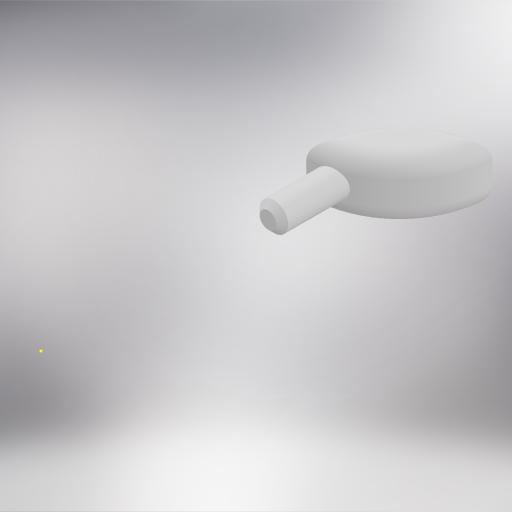
# Autodesk Inventor part: Apple_logo_red
Saved by Autodesk Inventor 2024 (Build 280153000, 153)
## iProperties
Created: 2023-10-30
Part Number: Apple_logo_red
Material: Generic
Document SubType Name: Modeling
Designer: SSAFY
Density: 1 g/cm^3
Appearance: Default
Author: SSAFY
Autodesk Inventor part; units mm, degrees
ref_plane "YZ Plane" through (0, 0, 0) normal (1, 0, 0) x (0, 1, 0)
ref_plane "XZ Plane" through (0, 0, 0) normal (0, 1, 0) x (-1, 0, 0)
ref_plane "XY Plane" through (0, 0, 0) normal (0, 0, 1) x (1, 0, 0)
sketch "Sketch2" plane through (0, 0, 0) normal (0, 1, 0) x (-1, 0, 0)
  line L0 (0, 0) -> (-15.3807, 0) construction
  line L1 (0, 12) -> (0, -86.6461) construction
  circle A0 centre (0, 0) radius 2
  circle A1 centre (-12, 0) radius 10
  circle A2 centre (-23.3137, -11.3137) radius 6
  circle A3 centre (-16, -32.0624) radius 16
  line L2 (-16, -48.0624) -> (0, -48.0624)
  line L3 (-12, 10) -> (0, 10)
  line L4 (-12, 0) -> (-23.3137, -11.3137)
  arc A4 (-19.5628, 6.5425) -> (-31.8772, -34.041) centre (19.8923, -27.5896) ccw
  line L5 (0, 0) -> (15.3807, 0) construction
  circle A5 centre (0, 0) radius 2
  circle A6 centre (12, 0) radius 10
  circle A7 centre (23.3137, -11.3137) radius 6
  circle A8 centre (16, -32.0624) radius 16
  line L6 (16, -48.0624) -> (0, -48.0624)
  line L7 (12, 10) -> (0, 10)
  line L8 (12, 0) -> (23.3137, -11.3137)
  arc A9 (31.8772, -34.041) -> (19.5628, 6.5425) centre (-19.8923, -27.5896) ccw
  arc A10 (10.7519, -47.1773) -> (0, -45.8341) centre (2.2238, -71.7388) ccw
  arc A11 (0, 6.9317) -> (7.2, 8.7727) centre (0, 21.9317) ccw
  arc A12 (0, -45.8341) -> (-10.7519, -47.1773) centre (-2.2238, -71.7388) ccw
  arc A13 (-7.2, 8.7727) -> (0, 6.9317) centre (0, 21.9317) ccw
  line L9 (-23.3137, -11.3137) -> (-58.3661, -46.3661)
  line L10 (-12, 0) -> (-38.3514, 26.3514)
  line L11 (10.1546, -70.2379) -> (-38.6751, -21.4081)
  circle A14 centre (-36.0416, -24.0416) radius 16
  circle A15 centre (-12.4253, -47.658) radius 16
  circle A16 centre (3.9792, -64.0624) radius 16
  line L12 (0, 10) -> (0, -48.0624)
  point P0 (3.5695, -48.0677)
  point P1 (-12.0156, -63.6527)
  point P2 (-7.2, 8.7727)
  point P3 (-29.0893, -9.6311)
  point P4 (-30.4093, -39.0175)
  point P5 (-10.7519, -47.1773)
  point P6 (-21.638, -17.075)
  point P7 (-21.3191, -16.9725)
  point P8 (-21.6324, -17.0866)
  point P9 (-29.075, -9.638)
  point P10 (-32.2772, -27.8061)
  point P11 (-31.5956, -28.4877)
  point P12 (0, -45.8341)
  point P13 (-28.9285, -9.1986)
  dimension "d0" = 4
  dimension "d1" = 20
  dimension "d2" = 12
  dimension "d3" = 32
  dimension "d4" = 135
  dimension "d6" = 26
  dimension "d7" = 15
  dimension "d8" = 90
  dimension "d12" = 34
  dimension "d13" = 32
  dimension "d14" = 32
  dimension "d15" = 32
  constraints: 26 end point, 24 point on circle, 17 centre point, 13 symmetric about line, 13 tangent, 11 point on line, 2 coincident, 2 collinear, 2 horizontal, 1 parallel, 1 vertical, 7 other
  measures "d0" diameter of A0
  measures "d1" diameter of A1
  measures "d2" diameter of A2
  measures "d3" diameter of A3
  measures "d4" angle of L4 L0
  measures "d6" radius of A10
  measures "d7" radius of A11
  measures "d8" angle of L10 L4
  measures "d12" distance between parallel lines of L10 L11
  measures "d13" diameter of A14
  measures "d14" diameter of A15
  measures "d15" diameter of A16
sketch "Sketch9" plane through (0, 0, 0) normal (0, 1, 0) x (-1, 0, 0)
  point P0 (0, 0)
extrude "Extrusion5" add sketch "Sketch2" along normal mid plane 10 contours A16 L11 A15 | A15 L11 A16
fillet "Fillet1" radius 3 4 edges at (7.3345, 5, -52.7487) (1.1116, 5, -58.9717) (7.3345, -5, -52.7487) (1.1116, -5, -58.9717)
sketch "Sketch11" plane through (0, 0, 0) normal (0, 1, 0) x (-1, 0, 0)
  line L0 (0, -51.9266) -> (-2.4, -51.9266)
  line L1 (-2.4, -51.9266) -> (-2.4, -38.0677)
  line L2 (-2.4, -38.0677) -> (0, -38.0677)
  line L3 (0, -38.0677) -> (0, -51.9266)
  arc A0 (-12.0156, -63.6527) -> (3.5695, -48.0677) centre (-12.4253, -47.658) ccw construction
  line L4 (3.5695, -48.0677) -> (-7.5617, -48.0677)
  point P0 (0, 0)
  dimension "d48" = 10
  dimension "d49" = 4.8
  dimension "d50" = 0
  constraints: 10 end point, 2 horizontal, 2 parallel, 1 perpendicular
  measures "d48" distance between parallel lines of L2 L4
  measures "d49" diameter of L1 L3
  measures "d50" distance from line of point (0, 0) L3
revolve "Revolution3" add sketch "Sketch11" angle 360 about axis through (0, 0, -38.0677) along (0, 0, -1)
chamfer "Chamfer5" distance 1 angle 45 1 edges at (-2.4, 0, -38.0677)
sketch "Sketch5" plane through (0, 0, 0) normal (0, 1, 0) x (-1, 0, 0)
  line L0 (-23.3137, -11.3137) -> (-58.3661, -46.3661) construction
  circle A0 centre (-36.0416, -24.0416) radius 16 projected
  line L1 (-36.0416, -24.0416) -> (-36.0416, 0)
  line L2 (0, 0) -> (0, -9.638)
  line L3 (-29.075, -9.638) -> (29.075, -9.638) construction
  line L4 (-36.0416, -24.0416) -> (-36.0416, -40.0416)
  point P0 (-36.0416, -8.0416)
  constraints: 6 end point, 2 vertical, 1 midpoint, 1 parallel, 1 point on circle, 1 point on line
sketch "Sketch6" plane through (0, 0, 0) normal (0, 1, 0) x (-1, 0, 0)
  line L0 (40.7884, -34.041) -> (-37.1762, -34.041)
  line L1 (-37.1762, -34.041) -> (-37.1762, -50.8727)
  line L2 (-37.1762, -50.8727) -> (40.7884, -50.8727)
  line L3 (40.7884, -50.8727) -> (40.7884, -34.041)
  point P0 (0, 0)
  dimension "d34" = 45
  dimension "d35" = 2
  constraints: 6 end point, 2 point on line, 2 vertical, 1 coincident, 1 other
  measures "d34" angle of L2 L0
  measures "d35" distance from line of point (-25.551, -34.041) L0
sketch "Sketch3" plane through (0, 0, 0) normal (0, -1, 0) x (1, 0, 0)
  line L0 (-51.3811, -10) -> (56.2604, -10)
  line L1 (56.2604, -10) -> (56.2604, -25)
  line L2 (56.2604, -25) -> (-51.3811, -25)
  line L3 (-51.3811, -25) -> (-51.3811, -10)
  point P0 (0, 0)
  dimension "d22" = 15
  dimension "d23" = 10
  constraints: 8 end point, 2 parallel, 1 horizontal, 1 perpendicular
  measures "d22" distance of L0.end L1.end
  measures "d23" distance from line of L0 point (0, 0)
body "Solid1"
body "Solid2"
body "Solid3"
